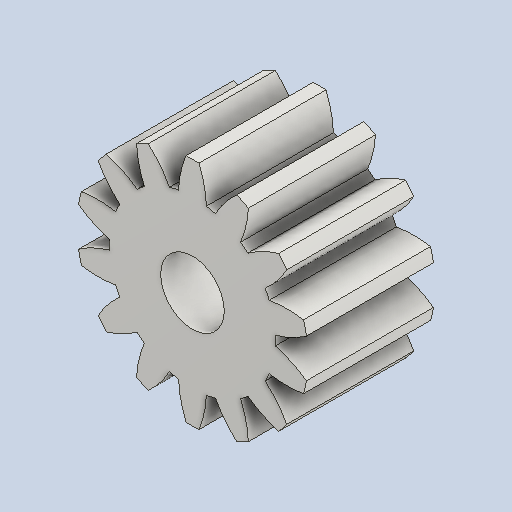
# Autodesk Inventor part: Spur Gear2
Saved by Autodesk Inventor 2022.3 (Build 263350000, 350)
## iProperties
CustomPartVersion: 1
Created: 2023-01-16
Part Number: Spur Gear2
Material: Steel
Document SubType Name: Modeling
Designer: komputer
Categories: <?xml version="1.0" encoding="UTF-16"?> <MemberInstance><Categories><FamilyTemplate><FamilyTemplateParameter ValueType="xs:double" Id="1" ObjectReferenceKey="da_z" ObjectType="kUserParameterObject"/><FamilyTemplateParameter ValueType="xs:double" Id="2" ObjectReferenceKey="da_b" ObjectType="kUserParameterObject"/><FamilyTemplateParameter ValueType="xs:double" Id="3" ObjectReferenceKey="da_beta" ObjectType="kUserParameterObject"/><FamilyTemplateParameter ValueType="xs:double" Id="4" ObjectReferenceKey="da_da" ObjectType="kUserParameterObject"/><FamilyTemplateParameter ValueType="xs:double" Id="5" ObjectReferenceKey="da_aw" ObjectType="kUserParameterObject"/><FamilyTemplateParameter ValueType="xs:string" Id="6" ObjectReferenceKey="EAIAABAAAACIAQAAAAAAAIAAAAAAAAAA" ObjectType="83910656" SubObjectId="SurfaceGeometry"/></FamilyTemplate><ParamToTemplateMap><ParamToTemplate CategoryParameter="//CategoryParameter[@InternalName='046C89C9-8512-4d59-83FE-43B91F4F132A']" TemplateParameter="1"/><ParamToTemplate CategoryParameter="//CategoryParameter[@InternalName='2552DF32-E462-4b46-AEBF-C6C7768E72AC']" TemplateParameter="2"/><ParamToTemplate CategoryParameter="//CategoryParameter[@InternalName='C9EE641D-15FC-4fae-A226-E94C4372FDD7']" TemplateParameter="3"/><ParamToTemplate><ParamToTemplate CategoryParameter="//CategoryParameter[@InternalName='00B6519A-459B-49c7-AD84-2E56D39A5744']" ConstantValue="0.000000"/></ParamToTemplate><ParamToTemplate><ParamToTemplate CategoryParameter="//CategoryParameter[@InternalName='04B31F0E-C7A6-4894-AA32-9629BEFACF47']" ConstantValue="1.000000"/></ParamToTemplate><ParamToTemplate><ParamToTemplate CategoryParameter="//CategoryParameter[@InternalName='43CBEC2E-7847-49e7-A936-2F7889FCB2D9']" ConstantValue="0.250000"/></ParamToTemplate><ParamToTemplate><ParamToTemplate CategoryParameter="//CategoryParameter[@InternalName='B1EFC894-105D-4ebd-86BF-FA20ED196853']" ConstantValue="0.350000"/></ParamToTemplate><ParamToTemplate><ParamToTemplate CategoryParameter="//CategoryParameter[@InternalName='51175063-3D10-4879-93E8-6246FE8B403D']" ConstantValue="2060000000.000000"/></ParamToTemplate><ParamToTemplate><ParamToTemplate CategoryParameter="//CategoryParameter[@InternalName='A3A52E27-4454-46a9-B0BD-C932399B70AF']" ConstantValue="0.300000"/></ParamToTemplate><ParamToTemplate><ParamToTemplate CategoryParameter="//CategoryParameter[@InternalName='91B76062-C214-41d9-B1B9-14D2AB99603D']" ConstantValue="0.045480"/></ParamToTemplate><ParamToTemplate><ParamToTemplate CategoryParameter="//CategoryParameter[@InternalName='374E806E-8B8A-4dda-A9AA-1039D6500AD2']" ConstantValue="21.987687"/></ParamToTemplate><ParamToTemplate><ParamToTemplate CategoryParameter="//CategoryParameter[@InternalName='2D373A89-B862-43d6-8D0B-0CBF12AB9F6C']" ConstantValue="0.349066"/></ParamToTemplate><ParamToTemplate CategoryParameter="//CategoryParameter[@InternalName='37777632-D6A2-4fac-9D53-DB8ACD95C989']" TemplateParameter="4"/><ParamToTemplate CategoryParameter="//CategoryParameter[@InternalName='FD1017F1-B727-4f7e-9707-0F86F1FF9423']" TemplateParameter="5"/><ParamToTemplate><ParamToTemplate CategoryParameter="//CategoryParameter[@InternalName='9E1B4470-B2D3-4ff1-B813-535BB4CDF51A']" ConstantValue="3520000.000000"/></ParamToTemplate><ParamToTemplate><ParamToTemplate CategoryParameter="//CategoryParameter[@InternalName='F8452263-BFF6-458c-9FB1-07C4B99E95CD']" ConstantValue="11400000.000000"/></ParamToTemplate><ParamToTemplate><ParamToTemplate CategoryParameter="//CategoryParameter[@InternalName='3E3BB259-FD49-497f-8171-6EBC954A3479']" ConstantValue="2.000000"/></ParamToTemplate><ParamToTemplate CategoryParameter="//CategoryParameter[@InternalName='27C3BAF2-7550-4e4b-AE2C-0DB134B7D9B7']" TemplateParameter="6"/></ParamToTemplateMap><Category DisplayName="Gear" InternalName="DC85795E-93AB-48d5-8EEE-5A27447B64BD" Mnemonic="Gear"><CategoryParameter DisplayName="z" InternalName="046C89C9-8512-4d59-83FE-43B91F4F132A" Mnemonic="z"/><CategoryParameter DisplayName="b" InternalName="2552DF32-E462-4b46-AEBF-C6C7768E72AC" Mnemonic="b"/><CategoryParameter DisplayName="||b|" InternalName="C9EE641D-15FC-4fae-A226-E94C4372FDD7" Mnemonic="beta"/><CategoryParameter DisplayName="x" InternalName="00B6519A-459B-49c7-AD84-2E56D39A5744" Mnemonic="x"/><CategoryParameter DisplayName="a*" InternalName="04B31F0E-C7A6-4894-AA32-9629BEFACF47" Mnemonic="a"/><CategoryParameter DisplayName="c*" InternalName="43CBEC2E-7847-49e7-A936-2F7889FCB2D9" Mnemonic="c"/><CategoryParameter DisplayName="r|.f|*" InternalName="B1EFC894-105D-4ebd-86BF-FA20ED196853" Mnemonic="rf"/><CategoryParameter DisplayName="E" InternalName="51175063-3D10-4879-93E8-6246FE8B403D" Mnemonic="E"/><CategoryParameter DisplayName="||m|" InternalName="A3A52E27-4454-46a9-B0BD-C932399B70AF" Mnemonic="mi"/><Category DisplayName="SpurGear" InternalName="26C5A22E-A91E-4dfd-A3B3-23CCAFAE1764" Mnemonic="SpurGear"><CategoryParameter DisplayName="m" InternalName="91B76062-C214-41d9-B1B9-14D2AB99603D" Mnemonic="m"/><CategoryParameter DisplayName="P" InternalName="374E806E-8B8A-4dda-A9AA-1039D6500AD2" Mnemonic="PP"/><CategoryParameter DisplayName="||a|" InternalName="2D373A89-B862-43d6-8D0B-0CBF12AB9F6C" Mnemonic="alpha"/><CategoryParameter DisplayName="d|.a|" InternalName="37777632-D6A2-4fac-9D53-DB8ACD95C989" Mnemonic="da"/><CategoryParameter DisplayName="a|.w|" InternalName="FD1017F1-B727-4f7e-9707-0F86F1FF9423" Mnemonic="aw"/><CategoryParameter DisplayName="||s||.Flim|" InternalName="9E1B4470-B2D3-4ff1-B813-535BB4CDF51A" Mnemonic="sFlim"/><CategoryParameter DisplayName="||s||.Hlim|" InternalName="F8452263-BFF6-458c-9FB1-07C4B99E95CD" Mnemonic="sHlim"/><CategoryParameter DisplayName="type" InternalName="3E3BB259-FD49-497f-8171-6EBC954A3479" Mnemonic="type"/><CategoryParameter DisplayName="PitchDiameter" InternalName="27C3BAF2-7550-4e4b-AE2C-0DB134B7D9B7" Mnemonic="IDS_PITCHDIAM"/></Category></Category></Categories></MemberInstance>
Density: 1 g/cm^3
Appearance: Steel
Author: komputer
Autodesk Inventor part; units mm, degrees
sketch "Sketch1" plane through (0, 0, 0) normal (0, 0, 1) x (1, 0, 0)
  circle A0 centre (0, 0) radius 3.6384
  dimension "d0" = 7.2768
  constraints: 1 centre point
  measures "d0" diameter of A0
extrude "Extrusion1" add sketch "Sketch1" along normal blind 20
ref_plane "Work Plane2" through (0, 0, 10) normal (0, 0, 1) x (1, 0, 0)
sketch "Sketch2" plane through (0, 0, 0) normal (0, 0, -1) x (-1, 0, 0)
  circle A0 centre (0, 0) radius 3.6384 projected
  circle A1 centre (0, 0) radius 3.1836
  dimension "d3" = 6.3672
  constraints: 1 centre point, 1 coincident
  measures "d3" diameter of A1
surface extrude "Pitch Diameter" sketch "Sketch2" against normal through all shown no curves A1
ref_plane "Work Plane8" through (0, 0, 0) normal (0.9749279, 0.2225209, 0) x (0, 0, 1)
ref_plane "Work Plane9" through (0, 0, 0) normal (1, 0, 0) x (0, 1, 0)
spur gear teeth "Spur Gear" teeth 14 pitch diameter 6.3672 tip diameter 7.2768 root diameter 5.2302 face width 20 start plane through (0, 0, 0) normal (0, 0, -1) x (-1, 0, 0)
sketch "Sketch3" plane through (0, 0, 20) normal (0, 0, 1) x (1, 0, 0)
  arc A0 (-1.76, 3.1844) -> (-1.5133, 2.1328) centre (1.3248, 3.3532) ccw projected
  arc A1 (-1.5133, 2.1328) -> (-1.7426, 1.9499) centre (0, 0) ccw projected
  arc A2 (-1.7426, 1.9499) -> (-2.7129, 2.4244) centre (-3.564, -0.5454) ccw projected
  arc A3 (-2.7129, 2.4244) -> (-2.9673, 2.1054) centre (0, 0) ccw projected
  arc A4 (-2.9673, 2.1054) -> (-2.2888, 1.265) centre (-0.2613, 3.596) ccw projected
  arc A5 (-2.2888, 1.265) -> (-2.416, 1.0008) centre (0, 0) ccw projected
  arc A6 (-2.416, 1.0008) -> (-3.4962, 1.0072) centre (-2.9744, -2.0378) ccw projected
  arc A7 (-3.4962, 1.0072) -> (-3.587, 0.6095) centre (0, 0) ccw projected
  arc A8 (-3.587, 0.6095) -> (-2.611, 0.1466) centre (-1.7957, 3.1265) ccw projected
  arc A9 (-2.611, 0.1466) -> (-2.611, -0.1466) centre (0, 0) ccw projected
  arc A10 (-2.611, -0.1466) -> (-3.587, -0.6095) centre (-1.7957, -3.1265) ccw projected
  arc A11 (-3.587, -0.6095) -> (-3.4962, -1.0072) centre (0, 0) ccw projected
  arc A12 (-3.4962, -1.0072) -> (-2.416, -1.0008) centre (-2.9744, 2.0378) ccw projected
  arc A13 (-2.416, -1.0008) -> (-2.2888, -1.265) centre (0, 0) ccw projected
  arc A14 (-2.2888, -1.265) -> (-2.9673, -2.1054) centre (-0.2613, -3.596) ccw projected
  arc A15 (-2.9673, -2.1054) -> (-2.7129, -2.4244) centre (0, 0) ccw projected
  arc A16 (-2.7129, -2.4244) -> (-1.7426, -1.9499) centre (-3.564, 0.5454) ccw projected
  arc A17 (-1.7426, -1.9499) -> (-1.5133, -2.1328) centre (0, 0) ccw projected
  arc A18 (-1.5133, -2.1328) -> (-1.76, -3.1844) centre (1.3248, -3.3532) ccw projected
  arc A19 (-1.76, -3.1844) -> (-1.3924, -3.3614) centre (0, 0) ccw projected
  arc A20 (-1.3924, -3.3614) -> (-0.724, -2.5129) centre (-3.4477, -1.0549) ccw projected
  arc A21 (-0.724, -2.5129) -> (-0.438, -2.5782) centre (0, 0) ccw projected
  arc A22 (-0.438, -2.5782) -> (-0.204, -3.6327) centre (2.6485, -2.4464) ccw projected
  arc A23 (-0.204, -3.6327) -> (0.204, -3.6327) centre (0, 0) ccw projected
  arc A24 (0.204, -3.6327) -> (0.438, -2.5782) centre (-2.6485, -2.4464) ccw projected
  arc A25 (0.438, -2.5782) -> (0.724, -2.5129) centre (0, 0) ccw projected
  arc A26 (0.724, -2.5129) -> (1.3924, -3.3614) centre (3.4477, -1.0549) ccw projected
  arc A27 (1.3924, -3.3614) -> (1.76, -3.1844) centre (0, 0) ccw projected
  arc A28 (1.76, -3.1844) -> (1.5133, -2.1328) centre (-1.3248, -3.3532) ccw projected
  arc A29 (1.5133, -2.1328) -> (1.7426, -1.9499) centre (0, 0) ccw projected
  arc A30 (1.7426, -1.9499) -> (2.7129, -2.4244) centre (3.564, 0.5454) ccw projected
  arc A31 (2.7129, -2.4244) -> (2.9673, -2.1054) centre (0, 0) ccw projected
  arc A32 (2.9673, -2.1054) -> (2.2888, -1.265) centre (0.2613, -3.596) ccw projected
  arc A33 (2.2888, -1.265) -> (2.416, -1.0008) centre (0, 0) ccw projected
  arc A34 (2.416, -1.0008) -> (3.4962, -1.0072) centre (2.9744, 2.0378) ccw projected
  arc A35 (3.4962, -1.0072) -> (3.587, -0.6095) centre (0, 0) ccw projected
  arc A36 (3.587, -0.6095) -> (2.611, -0.1466) centre (1.7957, -3.1265) ccw projected
  arc A37 (2.611, -0.1466) -> (2.611, 0.1466) centre (0, 0) ccw projected
  arc A38 (2.611, 0.1466) -> (3.587, 0.6095) centre (1.7957, 3.1265) ccw projected
  arc A39 (3.587, 0.6095) -> (3.4962, 1.0072) centre (0, 0) ccw projected
  arc A40 (3.4962, 1.0072) -> (2.416, 1.0008) centre (2.9744, -2.0378) ccw projected
  arc A41 (2.416, 1.0008) -> (2.2888, 1.265) centre (0, 0) ccw projected
  arc A42 (2.2888, 1.265) -> (2.9673, 2.1054) centre (0.2613, 3.596) ccw projected
  arc A43 (2.9673, 2.1054) -> (2.7129, 2.4244) centre (0, 0) ccw projected
  arc A44 (2.7129, 2.4244) -> (1.7426, 1.9499) centre (3.564, -0.5454) ccw projected
  arc A45 (1.7426, 1.9499) -> (1.5133, 2.1328) centre (0, 0) ccw projected
  arc A46 (1.5133, 2.1328) -> (1.76, 3.1844) centre (-1.3248, 3.3532) ccw projected
  arc A47 (1.76, 3.1844) -> (1.3924, 3.3614) centre (0, 0) ccw projected
  arc A48 (1.3924, 3.3614) -> (0.724, 2.5129) centre (3.4477, 1.0549) ccw projected
  arc A49 (0.724, 2.5129) -> (0.438, 2.5782) centre (0, 0) ccw projected
  arc A50 (0.438, 2.5782) -> (0.204, 3.6327) centre (-2.6485, 2.4464) ccw projected
  arc A51 (0.204, 3.6327) -> (-0.204, 3.6327) centre (0, 0) ccw projected
  arc A52 (-0.204, 3.6327) -> (-0.438, 2.5782) centre (2.6485, 2.4464) ccw projected
  arc A53 (-0.438, 2.5782) -> (-0.724, 2.5129) centre (0, 0) ccw projected
  arc A54 (-0.724, 2.5129) -> (-1.3924, 3.3614) centre (-3.4477, 1.0549) ccw projected
  arc A55 (-1.3924, 3.3614) -> (-1.76, 3.1844) centre (0, 0) ccw projected
extrude "Extrusion2" cut sketch "Sketch3" against normal blind 16
sketch "Sketch4" plane through (0, 0, 4) normal (0, 0, 1) x (1, 0, 0)
  circle A0 centre (0, 0) radius 1
  dimension "d51" = 2
  constraints: 1 centre point, 1 coincident
  measures "d51" diameter of A0
extrude "Extrusion3" cut sketch "Sketch4" against normal through all
equation "\"d0\" = da_da"
equation "\"d1\" = da_b"
equation "\"d3\" = da_d"
equation "\"d16\" = da_aw"
equation "\"d43\" = da_aw"
equation "\"d46\" = da_aw"
equation "\"da_da\" = 7.2768"
equation "\"da_b\" = 20"
equation "\"da_d\" = 6.3672"
equation "\"da_aw\" = 5.0028"
body "Solid1"
body "Srf1"
